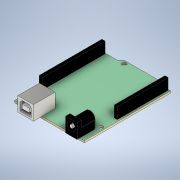
# Autodesk Inventor part: RoughArduino
Saved by Autodesk Inventor 2020 (Build 240168000, 168)
## iProperties
Created: 2023-02-03
Part Number: RoughArduino
Material: Generic
Document SubType Name: Modeling
Designer: legoo
Density: 1 g/cm^3
Appearance: Default
Author: legoo
Autodesk Inventor part; units mm, degrees
ref_plane "YZ Plane" through (0, 0, 0) normal (1, 0, 0) x (0, 1, 0)
ref_plane "XZ Plane" through (0, 0, 0) normal (0, 1, 0) x (-1, 0, 0)
ref_plane "XY Plane" through (0, 0, 0) normal (0, 0, 1) x (1, 0, 0)
sketch "Sketch1" plane through (0, 0, 0) normal (0, 1, 0) x (-1, 0, 0)
  line L0 (0, 0) -> (53.34, 0)
  line L1 (53.34, 0) -> (53.34, -66.04)
  line L2 (0, -66.04) -> (0, 0)
  circle A0 centre (50.8, -15.24) radius 1.6
  circle A1 centre (2.54, -15.24) radius 1.6
  circle A2 centre (35.56, -66.04) radius 1.6
  circle A3 centre (7.62, -66.04) radius 1.6
  line L3 (2.54, -66.04) -> (5.08, -68.58)
  line L4 (5.08, -68.58) -> (38.02, -68.58)
  line L5 (38.02, -68.58) -> (40.56, -66.04)
  line L6 (53.34, -66.04) -> (40.56, -66.04)
  line L7 (2.54, -66.04) -> (0, -66.04)
  dimension "d0" = 66.04
  dimension "d1" = 53.34
  dimension "d2" = 3.2
  dimension "d3" = 2.54
  dimension "d4" = 2.54
  dimension "d5" = 45.72
  dimension "d6" = 17.78
  dimension "d7" = 2.54
  dimension "d8" = 2.54
  dimension "d9" = 2.54
  dimension "d10" = 2.54
  dimension "d11" = 15.24
  dimension "d12" = 15.24
  dimension "d13" = 5
  constraints: 16 end point, 4 centre point, 3 equal radius, 3 parallel, 2 horizontal, 1 perpendicular
  measures "d0" distance of L0.end L1.end
  measures "d1" distance of L1.end L2.start
  measures "d2" diameter of A2
  measures "d3" distance from line of L1 A0.centre
  measures "d4" distance from line of L2 A1.centre
  measures "d5" distance from line of A3.centre L1
  measures "d6" distance from line of A2.centre L1
  measures "d7" distance from line of A2.centre L4
  measures "d8" horizontal distance of L4.end L5.end
  measures "d9" horizontal distance of L3.start L3.end
  measures "d10" distance of L2.start L3.start
  measures "d11" distance from line of L0 A0.centre
  measures "d12" distance from line of L0 A1.centre
  measures "d13" distance of A2.centre L5.end
extrude "Extrusion1" add sketch "Sketch1" along normal blind 1.5
sketch "Sketch2" plane through (0, 1.5, 0) normal (0, 1, 0) x (1, 0, 0)
  line L0 (-44.34, 10) -> (-32.34, 10)
  line L1 (-32.34, 10) -> (-32.34, -6.5)
  line L2 (-32.34, -6.5) -> (-44.34, -6.5)
  line L3 (-44.34, -6.5) -> (-44.34, 10)
  line L4 (-53.34, 0) -> (0, 0) projected
  line L5 (-53.34, 66.04) -> (-53.34, 0) projected
  dimension "d16" = 12
  dimension "d17" = 16.5
  dimension "d18" = 6.5
  dimension "d41" = 9
  constraints: 8 end point, 2 parallel, 1 horizontal, 1 perpendicular
  measures "d16" distance of L1.end L2.end
  measures "d17" distance of L2.end L0.start
  measures "d18" distance between parallel lines of L2 L4
  measures "d41" distance between parallel lines of L3 L5
extrude "Extrusion2" add sketch "Sketch2" along normal blind 11
sketch "Sketch3" plane through (-44.34, 1.5, 6.5) normal (0, 0, 1) x (1, 0, 0)
  line L0 (3.25, 7.025) -> (8.75, 7.025)
  line L1 (8.75, 7.025) -> (8.75, 3.975)
  line L2 (8.75, 3.975) -> (3.25, 3.975)
  line L3 (3.25, 3.975) -> (3.25, 7.025)
  line L4 (1.775, 1.61) -> (10.225, 1.61)
  line L5 (10.225, 1.61) -> (10.225, 7.775)
  line L6 (8.61, 9.39) -> (3.39, 9.39)
  line L7 (1.775, 7.775) -> (1.775, 1.61)
  line L8 (1.775, 7.775) -> (3.39, 9.39)
  line L9 (8.61, 9.39) -> (10.225, 7.775)
  line L10 (12, 0) -> (12, 11) projected
  line L11 (0, 11) -> (12, 11) projected
  point P0 (44.34, -1.5)
  dimension "d21" = 8.45
  dimension "d22" = 1.775
  dimension "d23" = 5.5
  dimension "d25" = 1.475
  dimension "d26" = 3.05
  dimension "d27" = 7.78
  dimension "d28" = 45
  dimension "d29" = 45
  dimension "d30" = 2.365
  dimension "d31" = 1.61
  dimension "d32" = 0.75
  constraints: 20 end point, 5 parallel, 2 horizontal, 2 perpendicular
  measures "d21" distance of L4.start L4.end
  measures "d22" distance between parallel lines of L5 L10
  measures "d23" distance of L0.start L0.end
  measures "d25" distance between parallel lines of L5 L1
  measures "d26" distance between parallel lines of L2 L0
  measures "d27" distance between parallel lines of L4 L6
  measures "d28" angle of L7 L8
  measures "d29" angle of L9 L5
  measures "d30" distance between parallel lines of L6 L0
  measures "d31" distance between parallel lines of L6 L11
  measures "d32" distance from line of L5.end L0
extrude "Extrusion3" cut sketch "Sketch3" against normal blind 11
sketch "Sketch4" plane through (0, 1.5, 0) normal (0, 1, 0) x (1, 0, 0)
  line L0 (-12.5, 12.3) -> (-3.5, 12.3)
  line L1 (-3.5, 12.3) -> (-3.5, -2)
  line L2 (-3.5, -2) -> (-12.5, -2)
  line L3 (-12.5, -2) -> (-12.5, 12.3)
  line L4 (-32.34, 0) -> (0, 0) projected
  line L5 (0, 0) -> (0, 66.04) projected
  dimension "d35" = 9
  dimension "d36" = 14.3
  dimension "d37" = 2
  dimension "d40" = 3.5
  constraints: 8 end point, 2 parallel, 1 horizontal, 1 perpendicular
  measures "d35" distance of L0.start L0.end
  measures "d36" distance of L2.end L0.start
  measures "d37" distance between parallel lines of L2 L4
  measures "d40" distance between parallel lines of L5 L1
extrude "Extrusion4" add sketch "Sketch4" along normal blind 11
sketch "Sketch5" plane through (-12.5, 1.5, 2) normal (0, 0, 1) x (1, 0, 0)
  circle A0 centre (4.5957, 6.5) radius 3.15
  line L0 (0, 0) -> (9, 0) projected
  circle A1 centre (4.5957, 6.5) radius 1.25
  point P0 (12.5, -1.5)
  dimension "d42" = 6.5
  dimension "d43" = 6.3
  dimension "d44" = 2.5
  constraints: 2 centre point, 1 coincident
  measures "d42" distance from line of L0 A0.centre
  measures "d43" diameter of A0
  measures "d44" diameter of A1
extrude "Extrusion5" cut sketch "Sketch5" against normal blind 11
sketch "Sketch6" plane through (-3.5, 1.5, -12.3) normal (0, 0, -1) x (-1, 0, 0)
  line L0 (-2.56, 0) -> (0.64, 0) projected
  line L1 (0.5, 0) -> (0.5, 6)
  line L2 (1.58, 0) -> (34.52, 0) projected
  line L3 (8.5, 0) -> (8.5, 6)
  arc A0 (8.5, 6) -> (0.5, 6) centre (4.5, 6) ccw
  line L4 (9, 0) -> (9, 11) projected
  line L5 (0, 11) -> (9, 11) projected
  line L6 (0, 0) -> (0, 11) projected
  line L7 (9, 0) -> (0, 0) projected
  line L8 (9, 0) -> (9, 11) projected
  line L9 (0, 11) -> (9, 11) projected
  line L10 (0, 0) -> (0, 11) projected
  point P0 (-3.5, -1.5)
  dimension "d47" = 8
  dimension "d48" = 8
  dimension "d49" = 0.5
  dimension "d50" = 1
  dimension "d51" = 4.5
  constraints: 4 end point, 2 point on circle, 2 point on line, 1 centre point, 1 perpendicular, 1 vertical
  measures "d47" diameter of A0
  measures "d48" distance between parallel lines of L1 L3
  measures "d49" distance between parallel lines of L4 L3
  measures "d50" distance edge to line of A0 L5
  measures "d51" distance from line of L4 A0.centre
extrude "Extrusion6" cut sketch "Sketch6" against normal blind 1 contours L6 L5 L4 L2 L3 A0 L1 L0
sketch "Sketch7" plane through (-3.5, 1.5, -11.3) normal (0, 0, -1) x (-1, 0, 0)
  arc A0 (8.5, 6) -> (0.5, 6) centre (4.5, 6) ccw projected
  arc A1 (8.5, 6) -> (0.5, 6) centre (4.5, 6) ccw projected
  line L0 (0.5, 6) -> (0, 6)
  line L1 (0, 0) -> (0, 11) projected
  line L2 (0, 6) -> (0, 11)
  line L3 (0, 11) -> (9, 11) projected
  line L4 (9, 11) -> (0, 11)
  line L5 (9, 11) -> (9, 6)
  line L6 (8.5, 0) -> (8.5, 6) projected
  line L7 (9, 6) -> (8.5, 6)
  point P0 (-3.5, -1.5)
  constraints: 10 end point, 3 perpendicular, 1 collinear, 1 horizontal, 1 point on line
extrude "Extrusion7" cut sketch "Sketch7" against normal blind 9.8
sketch "Sketch8" plane through (0, 1.5, 0) normal (0, 1, 0) x (1, 0, 0)
  line L0 (-3.79, 26.54) -> (-1.29, 26.54)
  line L1 (-1.29, 26.54) -> (-1.29, 65.54)
  line L2 (-1.29, 65.54) -> (-3.79, 65.54)
  line L3 (-3.79, 65.54) -> (-3.79, 26.54)
  line L4 (-52.05, 17.54) -> (-49.55, 17.54)
  line L5 (-49.55, 17.54) -> (-49.55, 65.54)
  line L6 (-49.55, 65.54) -> (-52.05, 65.54)
  line L7 (-52.05, 65.54) -> (-52.05, 17.54)
  circle A0 centre (-50.8, 15.24) radius 1.6 projected
  circle A1 centre (-2.54, 15.24) radius 1.6 projected
  line L8 (0, 66.04) -> (-2.54, 66.04) projected
  line L9 (-40.56, 66.04) -> (-53.34, 66.04) projected
  point P0 (0, 0)
  dimension "d56" = 2.5
  dimension "d57" = 2.5
  dimension "d58" = 39
  dimension "d59" = 48
  dimension "d60" = 1.25
  dimension "d61" = 1.25
  dimension "d62" = 0.5
  dimension "d63" = 0.5
  constraints: 16 end point, 4 parallel, 2 horizontal, 2 perpendicular
  measures "d56" distance of L5.end L6.end
  measures "d57" distance of L1.end L2.end
  measures "d58" distance of L2.end L0.start
  measures "d59" distance of L6.end L4.start
  measures "d60" distance from line of L7 A0.centre
  measures "d61" distance from line of A1.centre L3
  measures "d62" distance between parallel lines of L8 L2
  measures "d63" distance between parallel lines of L6 L9
extrude "Extrusion8" add sketch "Sketch8" along normal blind 8.5 contours L3 L2 L1 L0 | L7 L6 L5 L4
body "Solid1"
